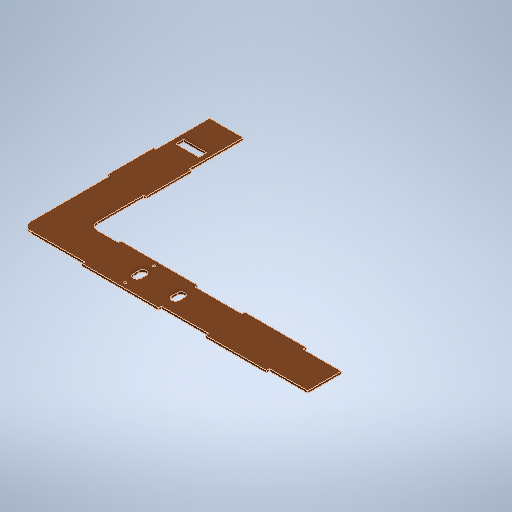
# Autodesk Inventor part: Path
Saved by Autodesk Inventor 2025.4 (Build 294407000, 407)
## iProperties
Created: 2026-04-10
Part Number: Path
Material: Generic
Document SubType Name: Sheet Metal
Designer: lenovo
Density: 1 g/cm^3
Sheet Metal Rule: Default_mm
Appearance: Default(1)
Author: lenovo
Autodesk Inventor part; units mm, degrees
ref_plane "YZ Plane" through (0, 0, 0) normal (1, 0, 0) x (0, 1, 0)
ref_plane "XZ Plane" through (0, 0, 0) normal (0, 1, 0) x (-1, 0, 0)
ref_plane "XY Plane" through (0, 0, 0) normal (0, 0, 1) x (1, 0, 0)
sketch "Sketch6" plane through (0, 1.5, 0) normal (0, 1, 0) x (1, 0, 0)
  line L0 (-131, 222) -> (-131, -12)
  line L1 (-131, 152) -> (-134, 152)
  line L2 (-134, 152) -> (-134, 92)
  line L3 (-134, 92) -> (-131, 92)
  line L4 (-131, 92) -> (-131, 152)
  line L5 (-87, 222) -> (-131, 222)
  line L6 (-109, 222) -> (-109, 171)
  line L7 (-124.04, 171) -> (-93.96, 171)
  line L8 (-87, 152) -> (-84, 152)
  line L9 (-84, 152) -> (-84, 92)
  line L10 (-84, 92) -> (-87, 92)
  line L11 (-87, 92) -> (-87, 152)
  point P0 (0, 0)
  point P1 (-134, 122)
  point P2 (-84, 122)
  dimension "d38" = 3
  dimension "d39" = 60
  dimension "d40" = 100
  measures "d38" distance of L3.end L2.end
  measures "d39" distance of L2.end L1.end
  measures "d40" distance from line of L5 point (-134, 122)
sketch "Sketch1" plane through (0, 0, 0) normal (0, 1, 0) x (-1, 0, 0)
  line L0 (-241, 22) -> (241, 22)
  line L1 (241, 22) -> (241, -22)
  line L2 (241, -22) -> (-241, -22)
  line L3 (-241, -22) -> (-241, 22)
  line L4 (-241, 22) -> (241, -22) construction
  line L5 (241, 22) -> (-241, -22) construction
  line L6 (50, -22) -> (-50, -22)
  line L7 (-50, -22) -> (-50, -25.5)
  line L8 (-50, -25.5) -> (50, -25.5)
  line L9 (50, -25.5) -> (50, -22)
  line L10 (50, -22) -> (-50, -25.5) construction
  line L11 (-50, -22) -> (50, -25.5) construction
  line L12 (241, 0) -> (-241, 0)
  line L13 (50, 22) -> (-50, 22)
  line L14 (-50, 22) -> (-50, 25.5)
  line L15 (-50, 25.5) -> (50, 25.5)
  line L16 (50, 25.5) -> (50, 22)
  line L17 (50, 22) -> (-50, 25.5) construction
  line L18 (-50, 22) -> (50, 25.5) construction
  line L19 (121, 15) -> (115.8, 15)
  line L20 (115.8, 15) -> (115.8, -15)
  line L21 (115.8, -15) -> (121, -15)
  line L22 (121, -15) -> (121, 15)
  line L23 (121, 15) -> (115.8, -15) construction
  line L24 (115.8, 15) -> (121, -15) construction
  circle A0 centre (0, -19) radius 1.6
  circle A1 centre (0, 19) radius 1.6
  line L25 (131, -22) -> (131, 22)
  point P0 (0, 0)
  point P1 (0, -23.75)
  point P2 (0, -22)
  point P3 (0, 23.75)
  point P4 (0, 22)
  point P5 (50, -22)
  point P6 (50, 22)
  point P7 (-50, 22)
  point P8 (-50, -22)
  point P9 (118.4, 0)
  point P10 (0, 0)
  dimension "d0" = 482
  dimension "d1" = 44
  dimension "d2" = 100
  dimension "d3" = 3.5
  dimension "d5" = 5.2
  dimension "d6" = 30
  dimension "d8" = 3.2
  dimension "d9" = 38
  dimension "d23" = 10
  dimension "d24" = 110
  measures "d0" distance of L1.end L2.end
  measures "d1" distance of L0.end L1.end
  measures "d2" distance of L8.end L7.end
  measures "d3" distance of L7.end L6.end
  measures "d5" distance of L21.end L20.end
  measures "d6" distance of L19.end L20.end
  measures "d8" diameter of A0
  measures "d9" diameter of A0.centre L12
  measures "d23" distance between parallel lines of L25 L22
  measures "d24" distance between parallel lines of L1 L25
extrude "Plate1" add sketch "Sketch1" along normal mid plane 3 contours L0 L25 L12 L22 L19 L20 L3 | L14 L15 L16 L0 | L12 L20 L21 L22 L25 L2 L3 | L20 L19 L22 L12 | L12 L22 L21 L20 | L2 L9 L8 L7
sketch "Sketch2" plane through (0, 1.5, 0) normal (0, 1, 0) x (1, 0, 0)
  line L0 (0, -3.5) -> (0, 3.5) construction
  line L1 (5, -3.5) -> (5, 3.5)
  line L2 (-5, 3.5) -> (-5, -3.5)
  arc A0 (-5, -3.5) -> (5, -3.5) centre (0, -3.5) ccw
  arc A1 (5, 3.5) -> (-5, 3.5) centre (0, 3.5) ccw
  line L3 (-50, -25.5) -> (50, -25.5) projected
  line L4 (25, -25.5) -> (25, 25.5)
  line L5 (50, 25.5) -> (-50, 25.5) projected
  circle A2 centre (0, -19) radius 1.6 projected
  line L6 (50, -3.5) -> (50, 3.5) construction
  line L7 (45, -3.5) -> (45, 3.5)
  line L8 (55, 3.5) -> (55, -3.5)
  arc A3 (45, -3.5) -> (55, -3.5) centre (50, -3.5) ccw
  arc A4 (55, 3.5) -> (45, 3.5) centre (50, 3.5) ccw
  point P0 (0, 0)
  point P1 (0, 8.5)
  point P2 (0, -8.5)
  point P3 (50, 0)
  point P4 (50, 8.5)
  point P5 (50, -8.5)
  dimension "d10" = 17
  dimension "d11" = 5
  dimension "d12" = 25
  constraints: 18 end point, 10 point on circle, 9 symmetric about line, 4 centre point, 4 tangent, 2 point on line, 2 vertical, 1 midpoint, 1 parallel, 2 other
  measures "d10" distance of point (0, 8.5) point (0, -8.5)
  measures "d11" radius of A1
  measures "d12" distance from line of A2.centre L4
extrude "Cut1" cut sketch "Sketch2" against normal blind 3 contours A0 L2 A1 L1 | L7 A4 L8 A3
sketch "Sketch3" plane through (0, 1.5, 0) normal (0, 1, 0) x (1, 0, 0)
  line L0 (-50, -25.5) -> (50, -25.5)
  line L1 (0, -25.5) -> (0, 25.5)
  line L2 (50, 25.5) -> (-50, 25.5)
  line L3 (-241, 0) -> (241, 0)
  line L4 (241, -22) -> (241, 22)
  line L5 (50, 22) -> (-50, 22)
  line L6 (191, 22) -> (111, 22)
  line L7 (111, 22) -> (111, 26)
  line L8 (111, 26) -> (191, 26)
  line L9 (191, 26) -> (191, 22)
  line L10 (191, -26) -> (191, -22)
  line L11 (191, -22) -> (111, -22)
  line L12 (111, -22) -> (111, -26)
  line L13 (111, -26) -> (191, -26)
  point P0 (0, 0)
  point P1 (151, 22)
  point P2 (151, -22)
sheet face with bend "Face2" sketch "Sketch3" thickness 3 toward (0, -1, 0) bend radius 3
bend "Bend1"
sketch "Sketch4" plane through (0, 1.5, 0) normal (0, 1, 0) x (1, 0, 0)
  line L0 (-50, 22) -> (-131, 22)
  line L1 (-131, 22) -> (-87, 22)
  line L2 (-87, 22) -> (-87, 222)
  line L3 (-87, 222) -> (-131, 222)
  line L4 (-131, 222) -> (-131, 22)
  point P0 (0, 0)
  dimension "d25" = 44
  dimension "d26" = 200
  measures "d25" distance between parallel lines of L4 L2
  measures "d26" distance of L3.end L0.end
sheet face with bend "Face3" sketch "Sketch4" thickness 3 toward (0, -1, 0) bend radius 3
bend "Bend2"
fillet "Corner Round1" radius 10 2 edges at (-87, 0, -22) (-131, 0, 22)
sketch "Sketch5" plane through (0, 1.5, 0) normal (0, 1, 0) x (1, 0, 0)
  line L0 (-124.04, 181) -> (-93.96, 181)
  line L1 (-93.96, 181) -> (-93.96, 171)
  line L2 (-93.96, 171) -> (-124.04, 171)
  line L3 (-124.04, 171) -> (-124.04, 181)
  line L4 (-87, 222) -> (-131, 222) projected
  point P0 (0, 0)
  point P1 (-109, 222)
  point P2 (-109, 181)
  dimension "d33" = 41
  dimension "d34" = 10
  dimension "d35" = 30.08
  constraints: 8 end point, 2 midpoint, 2 parallel, 1 horizontal, 1 perpendicular, 1 vertical alignment
  measures "d33" distance between parallel lines of L4 L0
  measures "d34" distance of L2.end L0.start
  measures "d35" distance between parallel lines of L3 L1
extrude "Cut2" cut sketch "Sketch5" against normal blind 3
sheet face with bend "Face4" sketch "Sketch6" thickness 3 toward (0, -1, 0) bend radius 3
bend "Bend3"
equation "\"d13\" = Thickness"
equation "\"d36\" = Thickness"
equation "\"d4\" = Thickness"
equation "\"d18\" = BendRadius"
equation "\"d19\" = BendReliefWidth"
equation "\"d21\" = MinimumRemnant"
equation "\"d20\" = BendReliefDepth"
equation "\"d22\" = TransitionRadius"
equation "\"d27\" = BendRadius"
equation "\"d28\" = BendReliefWidth"
equation "\"d30\" = MinimumRemnant"
equation "\"d29\" = BendReliefDepth"
equation "\"d31\" = TransitionRadius"
equation "\"d41\" = BendRadius"
equation "\"d42\" = BendReliefWidth"
equation "\"d44\" = MinimumRemnant"
equation "\"d43\" = BendReliefDepth"
equation "\"d45\" = TransitionRadius"
equation "\"BendRadius\" = Thickness"
equation "\"BendReliefWidth\" = Thickness"
equation "\"BendReliefDepth\" = 0.5 * Thickness"
equation "\"CornerReliefSize\" = 4 * Thickness"
equation "\"MinimumRemnant\" = 2 * Thickness"
equation "\"TransitionRadius\" = BendRadius"
equation "\"JacobiRadiusSize\" = BendRadius"
equation "\"GapSize\" = Thickness"
equation "\"Thickness\" = 3"
body "Solid1"
